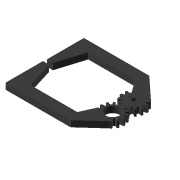
# Autodesk Inventor part: dientes mas afilados
Saved by Autodesk Inventor 2021 (Build 250183000, 183)
## iProperties
Created: 2022-06-07
Part Number: dientes mas afilados
Material: Genérico
Document SubType Name: Modeling
Designer: orgyn
Density: 1 g/cm^3
Appearance: Valor por defecto
Author: orgyn
Autodesk Inventor part; units mm, degrees
ref_plane "YZ Plane" through (0, 0, 0) normal (1, 0, 0) x (0, 1, 0)
ref_plane "XZ Plane" through (0, 0, 0) normal (0, 1, 0) x (-1, 0, 0)
ref_plane "XY Plane" through (0, 0, 0) normal (0, 0, 1) x (1, 0, 0)
sketch "Boceto1" plane through (0, 0, 0) normal (0, 1, 0) x (-1, 0, 0)
  circle A0 centre (0, 0) radius 4.5
  line L0 (7.4833, 0.4997) -> (5.4489, 0.7483)
  line L1 (7.4833, -0.4997) -> (5.4489, -0.7483)
  line L2 (6.5254, 3.6971) -> (4.5846, 3.0383)
  line L3 (6.9591, 2.7967) -> (5.2339, 1.69)
  line L4 (4.2751, 6.1623) -> (2.8123, 4.7266)
  line L5 (5.0565, 5.5391) -> (3.9823, 3.7936)
  line L6 (1.178, 7.4069) -> (0.483, 5.4788)
  line L7 (2.1524, 7.1845) -> (1.942, 5.1457)
  line L8 (-2.1524, 7.1845) -> (-1.942, 5.1457)
  line L9 (-1.178, 7.4069) -> (-0.483, 5.4788)
  line L10 (-5.0565, 5.5391) -> (-3.9823, 3.7936)
  line L11 (-4.2751, 6.1623) -> (-2.8123, 4.7266)
  line L12 (-6.9591, 2.7967) -> (-5.2339, 1.69)
  line L13 (-6.5254, 3.6971) -> (-4.5846, 3.0383)
  line L14 (-7.4833, -0.4997) -> (-5.4489, -0.7483)
  line L15 (-7.4833, 0.4997) -> (-5.4489, 0.7483)
  line L16 (-6.5254, -3.6971) -> (-4.5846, -3.0383)
  line L17 (-6.9591, -2.7967) -> (-5.2339, -1.69)
  line L18 (-4.2751, -6.1623) -> (-2.8123, -4.7266)
  line L19 (-5.0565, -5.5391) -> (-3.9823, -3.7936)
  line L20 (-1.178, -7.4069) -> (-0.483, -5.4788)
  line L21 (-2.1524, -7.1845) -> (-1.942, -5.1457)
  line L22 (2.1524, -7.1845) -> (1.942, -5.1457)
  line L23 (1.178, -7.4069) -> (0.483, -5.4788)
  line L24 (5.0565, -5.5391) -> (3.9823, -3.7936)
  line L25 (4.2751, -6.1623) -> (2.8123, -4.7266)
  line L26 (6.9591, -2.7967) -> (5.2339, -1.69)
  line L27 (6.5254, -3.6971) -> (4.5846, -3.0383)
  arc A1 (5.0565, 5.5391) -> (4.2751, 6.1623) centre (0, 0) ccw
  arc A2 (2.1524, 7.1845) -> (1.178, 7.4069) centre (0, 0) ccw
  arc A3 (-1.178, 7.4069) -> (-2.1524, 7.1845) centre (0, 0) ccw
  arc A4 (-4.2751, 6.1623) -> (-5.0565, 5.5391) centre (0, 0) ccw
  arc A5 (-6.5254, 3.6971) -> (-6.9591, 2.7967) centre (0, 0) ccw
  arc A6 (-7.4833, 0.4997) -> (-7.4833, -0.4997) centre (0, 0) ccw
  arc A7 (-6.9591, -2.7967) -> (-6.5254, -3.6971) centre (0, 0) ccw
  arc A8 (-5.0565, -5.5391) -> (-4.2751, -6.1623) centre (0, 0) ccw
  arc A9 (-2.1524, -7.1845) -> (-1.178, -7.4069) centre (0, 0) ccw
  arc A10 (1.178, -7.4069) -> (2.1524, -7.1845) centre (0, 0) ccw
  arc A11 (4.2751, -6.1623) -> (5.0565, -5.5391) centre (0, 0) ccw
  arc A12 (6.5254, -3.6971) -> (6.9591, -2.7967) centre (0, 0) ccw
  arc A13 (7.4833, -0.4997) -> (7.4833, 0.4997) centre (0, 0) ccw
  arc A14 (6.9591, 2.7967) -> (6.5254, 3.6971) centre (0, 0) ccw
  arc A15 (5.4489, 0.7483) -> (5.2339, 1.69) centre (0, 0) ccw
  arc A16 (4.5846, 3.0383) -> (3.9823, 3.7936) centre (0, 0) ccw
  arc A17 (5.2339, -1.69) -> (5.358, -1.2419) centre (0, 0) ccw
  arc A18 (5.358, 1.2419) -> (5.2339, 1.69) centre (0, 0) ccw
  arc A19 (4.5846, 3.0383) -> (3.9823, 3.7936) centre (0, 0) ccw
  arc A20 (2.8123, 4.7266) -> (1.942, 5.1457) centre (0, 0) ccw
  arc A21 (2.8123, 4.7266) -> (1.942, 5.1457) centre (0, 0) ccw
  arc A22 (0.483, 5.4788) -> (-0.483, 5.4788) centre (0, 0) ccw
  arc A23 (0.483, 5.4788) -> (-0.483, 5.4788) centre (0, 0) ccw
  arc A24 (-1.942, 5.1457) -> (-2.8123, 4.7266) centre (0, 0) ccw
  arc A25 (-1.942, 5.1457) -> (-2.8123, 4.7266) centre (0, 0) ccw
  arc A26 (-3.9823, 3.7936) -> (-4.5846, 3.0383) centre (0, 0) ccw
  arc A27 (-3.9823, 3.7936) -> (-4.5846, 3.0383) centre (0, 0) ccw
  arc A28 (-5.2339, 1.69) -> (-5.4489, 0.7483) centre (0, 0) ccw
  arc A29 (-5.2339, 1.69) -> (-5.4489, 0.7483) centre (0, 0) ccw
  arc A30 (-5.4489, -0.7483) -> (-5.2339, -1.69) centre (0, 0) ccw
  arc A31 (-5.4489, -0.7483) -> (-5.2339, -1.69) centre (0, 0) ccw
  arc A32 (-4.5846, -3.0383) -> (-3.9823, -3.7936) centre (0, 0) ccw
  arc A33 (-4.5846, -3.0383) -> (-3.9823, -3.7936) centre (0, 0) ccw
  arc A34 (-2.8123, -4.7266) -> (-1.942, -5.1457) centre (0, 0) ccw
  arc A35 (-2.8123, -4.7266) -> (-1.942, -5.1457) centre (0, 0) ccw
  arc A36 (-0.483, -5.4788) -> (0.483, -5.4788) centre (0, 0) ccw
  arc A37 (-0.483, -5.4788) -> (0.483, -5.4788) centre (0, 0) ccw
  arc A38 (1.942, -5.1457) -> (2.8123, -4.7266) centre (0, 0) ccw
  arc A39 (1.942, -5.1457) -> (2.8123, -4.7266) centre (0, 0) ccw
  arc A40 (3.9823, -3.7936) -> (4.5846, -3.0383) centre (0, 0) ccw
  arc A41 (3.9823, -3.7936) -> (4.5846, -3.0383) centre (0, 0) ccw
  arc A42 (5.2339, -1.69) -> (5.4489, -0.7483) centre (0, 0) ccw
  line L28 (0, 0) -> (0, 10.0549)
  line L29 (8.723, 17.9975) -> (50, 17.9975)
  line L30 (40.9223, 11.63) -> (10.9223, 11.63)
  line L31 (10.9223, 11.63) -> (4.3001, 3.4292)
  arc A43 (7.1491, -12.6497) -> (6.9755, -11.6654) centre (-0.3073, -13.457) ccw
  arc A44 (6.0604, -9.4944) -> (5.477, -8.6829) centre (-0.3073, -13.457) ccw
  line L32 (5.477, -8.6829) -> (3.68, -9.6687)
  line L33 (6.0604, -9.4944) -> (4.5536, -10.8838)
  line L34 (6.9755, -11.6654) -> (4.9288, -11.7739)
  circle A45 centre (-0.3073, -13.457) radius 4.5
  arc A46 (3.7105, -7.124) -> (2.8327, -6.646) centre (-0.3073, -13.457) ccw
  arc A47 (4.7536, -11.3036) -> (4.5536, -10.8838) centre (-0.3073, -13.457) ccw
  arc A48 (4.9288, -11.7739) -> (4.5536, -10.8838) centre (-0.3073, -13.457) ccw
  arc A49 (3.68, -9.6687) -> (2.9557, -9.0295) centre (-0.3073, -13.457) ccw
  arc A50 (3.68, -9.6687) -> (2.9557, -9.0295) centre (-0.3073, -13.457) ccw
  line L35 (3.7105, -7.124) -> (2.9557, -9.0295)
  line L36 (2.8327, -6.646) -> (1.6415, -8.3138)
  arc A51 (1.6415, -8.3138) -> (0.7116, -8.0522) centre (-0.3073, -13.457) ccw
  arc A52 (1.6415, -8.3138) -> (0.7116, -8.0522) centre (-0.3073, -13.457) ccw
  line L37 (0.5648, -6.0079) -> (0.7116, -8.0522)
  line L38 (-0.4334, -5.9581) -> (-0.7831, -7.9776)
  arc A53 (-0.7831, -7.9776) -> (-1.7344, -8.1453) centre (-0.3073, -13.457) ccw
  arc A54 (-0.7831, -7.9776) -> (-1.7344, -8.1453) centre (-0.3073, -13.457) ccw
  arc A55 (0.5648, -6.0079) -> (-0.4334, -5.9581) centre (-0.3073, -13.457) ccw
  arc A56 (4.2732, -16.5014) -> (4.7352, -15.6531) centre (-0.3073, -13.457) ccw
  arc A57 (4.2732, -16.5014) -> (4.7352, -15.6531) centre (-0.3073, -13.457) ccw
  arc A58 (4.9729, -18.7833) -> (5.6342, -18.0339) centre (-0.3073, -13.457) ccw
  arc A59 (6.761, -15.9648) -> (7.0316, -15.0027) centre (-0.3073, -13.457) ccw
  line L39 (4.9729, -18.7833) -> (3.283, -17.6235)
  line L40 (5.6342, -18.0339) -> (4.2732, -16.5014)
  arc A60 (5.1405, -14.2125) -> (5.1849, -13.7496) centre (-0.3073, -13.457) ccw
  arc A61 (5.1405, -14.2125) -> (5.1887, -13.2477) centre (-0.3073, -13.457) ccw
  line L41 (7.0316, -15.0027) -> (5.1405, -14.2125)
  line L42 (6.761, -15.9648) -> (4.7352, -15.6531)
  line L43 (7.1491, -12.6497) -> (5.1887, -13.2477)
  line L44 (-7.3756, -10.9492) -> (-5.3499, -11.2609)
  arc A62 (-4.8879, -10.4126) -> (-5.3499, -11.2609) centre (-0.3073, -13.457) ccw
  arc A63 (-4.8879, -10.4126) -> (-5.3499, -11.2609) centre (-0.3073, -13.457) ccw
  line L45 (-6.2489, -8.8801) -> (-4.8879, -10.4126)
  arc A64 (-3.1134, -8.7266) -> (-3.8977, -9.2905) centre (-0.3073, -13.457) ccw
  arc A65 (-3.1134, -8.7266) -> (-3.8977, -9.2905) centre (-0.3073, -13.457) ccw
  line L46 (-5.5875, -8.1307) -> (-3.8977, -9.2905)
  arc A66 (-5.5875, -8.1307) -> (-6.2489, -8.8801) centre (-0.3073, -13.457) ccw
  arc A67 (-5.7552, -12.7015) -> (-5.8034, -13.6663) centre (-0.3073, -13.457) ccw
  arc A68 (-5.7552, -12.7015) -> (-5.8034, -13.6663) centre (-0.3073, -13.457) ccw
  arc A69 (-7.3756, -10.9492) -> (-7.6463, -11.9112) centre (-0.3073, -13.457) ccw
  line L47 (-7.6463, -11.9112) -> (-5.7552, -12.7015)
  arc A70 (-5.5435, -15.1401) -> (-5.1683, -16.0302) centre (-0.3073, -13.457) ccw
  arc A71 (-5.5435, -15.1401) -> (-5.1683, -16.0302) centre (-0.3073, -13.457) ccw
  line L48 (-7.7638, -14.2643) -> (-5.8034, -13.6663)
  line L49 (-7.5902, -15.2486) -> (-5.5435, -15.1401)
  line L50 (-6.6751, -17.4196) -> (-5.1683, -16.0302)
  line L51 (-6.0916, -18.2311) -> (-4.2947, -17.2453)
  arc A72 (-6.6751, -17.4196) -> (-6.0916, -18.2311) centre (-0.3073, -13.457) ccw
  line L52 (-4.3251, -19.79) -> (-3.5704, -17.8844)
  arc A73 (-4.3251, -19.79) -> (-3.4474, -20.268) centre (-0.3073, -13.457) ccw
  arc A74 (-2.2561, -18.6002) -> (-1.3263, -18.8618) centre (-0.3073, -13.457) ccw
  arc A75 (-2.2561, -18.6002) -> (-1.3263, -18.8618) centre (-0.3073, -13.457) ccw
  arc A76 (0.1684, -18.9364) -> (1.1197, -18.7686) centre (-0.3073, -13.457) ccw
  arc A77 (0.1684, -18.9364) -> (1.1197, -18.7686) centre (-0.3073, -13.457) ccw
  line L53 (2.139, -20.5468) -> (1.1197, -18.7686)
  line L54 (-3.4474, -20.268) -> (-2.2561, -18.6002)
  arc A78 (-2.7536, -6.3672) -> (-3.6746, -6.7554) centre (-0.3073, -13.457) ccw
  line L55 (-2.7536, -6.3672) -> (-1.7344, -8.1453)
  line L56 (-3.6746, -6.7554) -> (-3.1134, -8.7266)
  arc A79 (2.4987, -18.1873) -> (3.283, -17.6235) centre (-0.3073, -13.457) ccw
  arc A80 (2.139, -20.5468) -> (3.0599, -20.1586) centre (-0.3073, -13.457) ccw
  line L57 (3.0599, -20.1586) -> (2.4987, -18.1873)
  arc A81 (2.4987, -18.1873) -> (3.283, -17.6235) centre (-0.3073, -13.457) ccw
  line L58 (-0.1813, -20.9559) -> (0.1684, -18.9364)
  arc A82 (-1.1795, -20.9061) -> (-0.1813, -20.9559) centre (-0.3073, -13.457) ccw
  line L59 (-1.1795, -20.9061) -> (-1.3263, -18.8618)
  arc A83 (-4.2947, -17.2453) -> (-3.5704, -17.8844) centre (-0.3073, -13.457) ccw
  arc A84 (-4.2947, -17.2453) -> (-3.5704, -17.8844) centre (-0.3073, -13.457) ccw
  line L60 (40.615, -25.087) -> (10.615, -25.087)
  line L61 (-7.7638, -14.2643) -> (-7.5902, -15.2486)
  line L62 (46.202, -5.6) -> (50, -5.6)
  line L63 (45.8947, -7.857) -> (49.6927, -7.857)
  line L64 (40.9223, 11.63) -> (46.202, -5.6)
  line L65 (45.8947, -7.857) -> (40.615, -25.087)
  line L66 (8.723, 17.9975) -> (-4.2751, 6.1623)
  line L67 (50, -5.6) -> (50, 17.9975)
  line L68 (10.615, -31.387) -> (40.615, -31.387)
  line L69 (40.615, -31.387) -> (49.6927, -31.387)
  line L70 (10.615, -31.387) -> (8.1024, -31.387)
  line L71 (10.615, -25.087) -> (4.2732, -16.5014)
  line L72 (8.1024, -31.387) -> (-6.0916, -18.2311)
  line L73 (10.9223, 11.63) -> (6.9591, 2.7967)
  circle A85 centre (-0.3073, -13.457) radius 1.5
  line L74 (49.6927, -7.857) -> (49.6927, -31.387)
  point P0 (5.1849, -13.7496)
  point P1 (4.7536, -11.3036)
  point P2 (5.358, -1.2419)
  dimension "d1" = 9
  dimension "d11" = 360
  dimension "d16" = 20
  dimension "d19" = 30
  dimension "d30" = 6.3
  dimension "d31" = 3
  constraints: 167 point on circle, 150 end point, 86 centre point, 7 coincident, 3 point on line, 2 perpendicular, 2 vertical, 1 horizontal, 85 other
  measures "d1" diameter of A0
  measures "d16" distance of L28.start L29.start
  measures "d19" distance of L30.start L30.end
  measures "d30" distance of L60.end L68.start
  measures "d31" diameter of A85
extrude "Extrusión1" add sketch "Boceto1" along normal blind 4 contours A22 L6 A2 L7 A20 L4 A1 L5 A16 L2 A14 L3 A15 L0 A13 L1 A42 A17 L26 A12 L27 A40 L24 A11 L25 A38 L22 A10 L23 A36 L20 A9 L21 A34 L18 A8 L19 A32 L16 A7 L17 A30 L14 A6 L15 A28 L12 A5 L13 A26 L10 A4 L11 A24 L8 A3 L9 | A22 L9 A3 L8 A24 L11 L66 L28 | L28 L66 L29 L67 L62 L64 L30 L31 A16 L5 A1 L4 A20 L7 A2 L6 A22 | L73 A14 L2 A16 L31 | L43 A61 A60 L41 A59 L42 A56 L71 A58 L39 A79 L57 A80 L53 A76 L58 A82 L59 A74 L54 A73 L52 A83 L51 A72 L50 A70 L49 L61 L48 A67 L47 A69 L44 A62 L45 A66 L46 A64 L56 A78 L55 A53 L38 A55 L37 A51 L36 A46 L35 A49 L32 A44 L33 A47 A48 L34 A43 | L71 L60 L65 L63 L74 L69 L68 L70 L72 L51 A83 L52 A73 L54 A74 L59 A82 L58 A76 L53 A80 L57 A79 L39 A58 | A45
